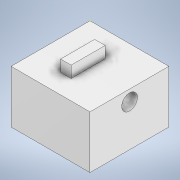
# Autodesk Inventor part: water tank 1
Saved by Autodesk Inventor 2022 (Build 260153000, 153)
## iProperties
Created: 2022-06-23
Part Number: water tank 1
Material: PVC, Unplasticized
Document SubType Name: Modeling
Designer: HP
Density: 1.29 g/cm^3
Appearance: Smooth - White
Author: HP
Autodesk Inventor part; units mm, degrees
ref_plane "YZ Plane" through (0, 0, 0) normal (1, 0, 0) x (0, 1, 0)
ref_plane "XZ Plane" through (0, 0, 0) normal (0, 1, 0) x (-1, 0, 0)
ref_plane "XY Plane" through (0, 0, 0) normal (0, 0, 1) x (1, 0, 0)
sketch "Sketch1" plane through (0, 0, 0) normal (0, 1, 0) x (-1, 0, 0)
  point P0 (0, 0)
sketch "Sketch2" plane through (0, 0, 0) normal (0, 0, 1) x (1, 0, 0)
  line L0 (0, 0) -> (150, 0)
  line L1 (150, 0) -> (150, -100)
  line L2 (150, -100) -> (0, -100)
  line L3 (0, -100) -> (0, 0)
  constraints: 8 end point, 2 parallel, 1 horizontal, 1 perpendicular
extrude "Extrusion1" add sketch "Sketch2" along normal blind 150
sketch "Sketch3" plane through (150, -100, 0) normal (1, 0, 0) x (0, 0, -1)
  circle A0 centre (-74.7614, 78.8048) radius 15
  point P0 (0, 100)
  dimension "d4" = 30
  constraints: 1 centre point
  measures "d4" diameter of A0
extrude "Extrusion2" cut sketch "Sketch3" against normal blind 40.75
sketch "Sketch4" plane through (0, 0, 0) normal (0, 1, 0) x (1, 0, 0)
  line L0 (57.0345, -48.171) -> (77.0345, -48.171)
  line L1 (77.0345, -48.171) -> (77.0345, -112.9129)
  line L2 (77.0345, -112.9129) -> (57.0345, -112.9129)
  line L3 (57.0345, -112.9129) -> (57.0345, -48.171)
  point P0 (0, 0)
  constraints: 8 end point, 2 parallel, 1 horizontal, 1 perpendicular
extrude "Extrusion3" add sketch "Sketch4" along normal blind 22
body "Solid1"
